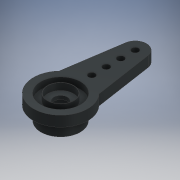
# Autodesk Inventor part: Servomotor-1
Saved by Autodesk Inventor 2019 (Build 230136000, 136)
## iProperties
Created: 2019-10-22
Part Number: Servomotor-1
Material: Generic
Document SubType Name: Modeling
Designer: User
Density: 1 g/cm^3
Appearance: Default
Mass: 0.43687 g
Surface Area: 7.91719 cm^2
Volume: 0.43687 cm^3
Author: User
Autodesk Inventor part; units mm, degrees
ref_plane "YZ Plane" through (0, 0, 0) normal (1, 0, 0) x (0, 1, 0)
ref_plane "XZ Plane" through (0, 0, 0) normal (0, 1, 0) x (-1, 0, 0)
ref_plane "XY Plane" through (0, 0, 0) normal (0, 0, 1) x (1, 0, 0)
sketch "Sketch1" plane through (0, 0, 0) normal (0, 0, 1) x (1, 0, 0)
  circle A0 centre (0, 0) radius 4.35
  dimension "d0" = 8.7
  constraints: 1 centre point, 1 coincident
  measures "d0" diameter of A0
extrude "Extrusion1" add sketch "Sketch1" along normal blind 3
sketch "Sketch2" plane through (0, 0, 0) normal (0, 0, -1) x (-1, 0, 0)
  circle A0 centre (0, 0) radius 3
  dimension "d3" = 6
  constraints: 1 centre point, 1 coincident
  measures "d3" diameter of A0
extrude "Extrusion2" cut sketch "Sketch2" against normal up to next
sketch "Sketch3" plane through (0, 0, 3) normal (0, 0, 1) x (1, 0, 0)
  arc A0 (2.4721, 16.8725) -> (-2.4721, 16.8725) centre (0, 16.5) ccw
  line L0 (-4.4, 4.0792) -> (-2.4721, 16.8725)
  line L1 (4.4, 4.0792) -> (2.4721, 16.8725)
  circle A1 centre (0, 16.5) radius 0.75
  circle A2 centre (0, 13.3) radius 0.75
  circle A3 centre (0, 10.1) radius 0.75
  circle A4 centre (0, 6.9) radius 0.75
  arc A5 (-4.4, 4.0792) -> (-4.4, -4.0792) centre (0, 0) ccw
  arc A6 (4.4, -4.0792) -> (4.4, 4.0792) centre (0, 0) ccw
  arc A7 (-4.4, -4.0792) -> (4.4, -4.0792) centre (0, 0) ccw
  line L2 (0, 6.9) -> (0, 4.35) construction
  circle A8 centre (0, 0) radius 4.35 construction
  dimension "d8" = 8.8
  dimension "d10" = 1.5
  dimension "d13" = 1.5
  dimension "d14" = 1.5
  dimension "d15" = 1.5
  constraints: 8 centre point, 8 point on circle, 6 end point, 2 coincident, 2 tangent, 1 vertical, 1 vertical alignment, 1 other
  measures "d8" distance of L0.start L1.start
  measures "d10" diameter of A1
  measures "d13" diameter of A2
  measures "d14" diameter of A3
  measures "d15" diameter of A4
extrude "Extrusion3" add sketch "Sketch3" along normal blind 2.3
sketch "Sketch4" plane through (0, 0, 5.3) normal (0, 0, 1) x (1, 0, 0)
  circle A0 centre (0, 0) radius 2.85
  circle A1 centre (0, 0) radius 4.4
  circle A2 centre (0, 0) radius 2.95
  dimension "d22" = 5.7
  dimension "d23" = 8.8
  dimension "d24" = 5.9
  constraints: 3 centre point, 3 coincident
  measures "d22" diameter of A0
  measures "d23" diameter of A1
  measures "d24" diameter of A2
extrude "Extrusion4" cut sketch "Sketch4" against normal blind 1.5
sketch "Sketch5" plane through (0, 0, 3.8) normal (0, 0, 1) x (1, 0, 0)
  circle A0 centre (0, 0) radius 1.5
  dimension "d27" = 3
  constraints: 1 centre point, 1 coincident
  measures "d27" diameter of A0
extrude "Extrusion5" cut sketch "Sketch5" against normal up to next
body "Solid1"
